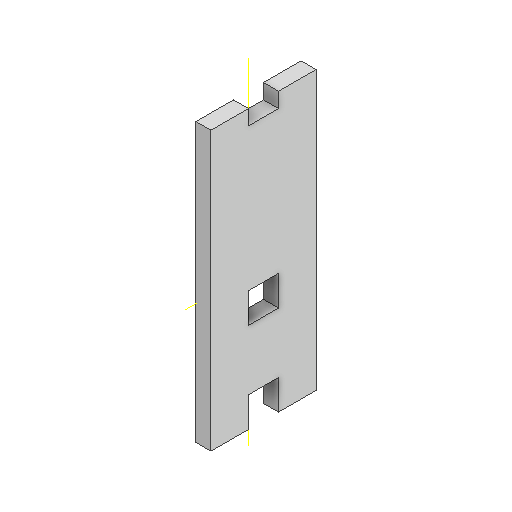
# Autodesk Inventor part: 분류대_COLUMN
Saved by Autodesk Inventor 2027 (Build 310192000, 192)
## iProperties
Created: 2026-09-17
Part Number: 분류대_COLUMN
Material: 일반
Document SubType Name: Modeling
Designer: User
Density: 1 g/cm^3
Appearance: 기본값
Author: User
Autodesk Inventor part; units mm, degrees
ref_plane "YZ 평면_우측면도" through (0, 0, 0) normal (1, 0, 0) x (0, 1, 0)
ref_plane "XZ 평면_평면도" through (0, 0, 0) normal (0, 1, 0) x (-1, 0, 0)
ref_plane "XY 평면_정면도" through (0, 0, 0) normal (0, 0, 1) x (1, 0, 0)
sketch "스케치1" plane through (0, 0, 0) normal (1, 0, 0) x (0, 1, 0)
  line L0 (-80, -35) -> (105, -35)
  line L1 (105, 35) -> (-80, 35)
  line L2 (95, -10) -> (105, -10)
  line L3 (105, 10) -> (95, 10)
  line L4 (95, 10) -> (95, -10)
  line L5 (105, -35) -> (105, -10)
  line L6 (105, 10) -> (105, 35)
  line L7 (-134, 0) -> (244, 0) projected
  line L8 (95, 10) -> (0, 10) construction
  line L9 (95, 10) -> (190, 10) construction
  line L10 (0, 10) -> (-20, 10)
  line L11 (-20, 10) -> (-20, -10)
  line L12 (-20, -10) -> (0, -10)
  line L13 (0, -10) -> (0, 10)
  line L14 (-60, 10) -> (-80, 10)
  line L15 (-80, -10) -> (-60, -10)
  line L16 (-60, -10) -> (-60, 10)
  line L17 (-80, 35) -> (-80, 10)
  line L18 (-80, -10) -> (-80, -35)
  line L19 (0, -49) -> (0, 49) projected
  point P0 (0, 0)
  dimension "d0" = 185
  dimension "d1" = 70
  dimension "d4" = 20
  dimension "d5" = 10
  dimension "d6" = 95
  dimension "d8" = 20
  dimension "d9" = 20
  dimension "d12" = 20
  dimension "d13" = 20
  dimension "d14" = 25
  dimension "d15" = 25
  dimension "d16" = 40
  constraints: 36 end point, 9 parallel, 6 horizontal, 3 perpendicular, 2 collinear, 2 other
  measures "d0" distance of L1.end L1.start
  measures "d1" distance of L1.start L0.end
  measures "d4" distance between parallel lines of L2 L3
  measures "d5" distance between parallel lines of L4 L5
  measures "d6" distance of L3.end L8.end
  measures "d8" distance of L12.end L11.end
  measures "d9" distance of L11.end L10.end
  measures "d12" distance between parallel lines of L15 L14
  measures "d13" distance between parallel lines of L18 L16
  measures "d14" distance between parallel lines of L10 L1
  measures "d15" distance between parallel lines of L0 L12
  measures "d16" distance between parallel lines of L16 L11
extrude "돌출1" add sketch "스케치1" along normal blind 10 contours L18 L15 L16 L7 L11 L12 L19 L0 | L19 L13 L7 L4 L2 L5 L0 | L13 L19 L1 L6 L3 L4 L7 | L16 L14 L17 L1 L19 L10 L11 L7
